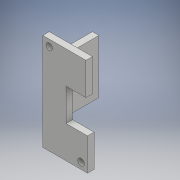
# Autodesk Inventor part: support-srf04
Saved by Autodesk Inventor 2017 (Build 210142000, 142)
## iProperties
Created: 2017-04-21
Part Number: support-srf04
Material: Generic
Document SubType Name: Modeling
Designer: franc
Density: 1 g/cm^3
Appearance: Default
Author: franc
Autodesk Inventor part; units mm, degrees
ref_plane "YZ Plane" through (0, 0, 0) normal (1, 0, 0) x (0, 1, 0)
ref_plane "XZ Plane" through (0, 0, 0) normal (0, 1, 0) x (-1, 0, 0)
ref_plane "XY Plane" through (0, 0, 0) normal (0, 0, 1) x (1, 0, 0)
sketch "Sketch1" plane through (0, 0, 0) normal (0, 1, 0) x (-1, 0, 0)
  line L0 (-9.1925, 10.3416) -> (10.8075, 10.3416)
  line L1 (10.8075, 10.3416) -> (10.8075, -34.6584)
  line L2 (10.8075, -34.6584) -> (-9.9379, -34.6584)
  line L3 (-9.9379, -34.6584) -> (-9.9379, -19.6584)
  line L4 (-9.1925, 10.3416) -> (-9.1925, -4.6584)
  line L5 (-9.1925, -4.6584) -> (0.0621, -4.6584)
  line L6 (0.0621, -4.6584) -> (0.0621, -19.6584)
  line L7 (0.0621, -19.6584) -> (-9.9379, -19.6584)
  circle A0 centre (-6.9379, -31.6584) radius 1.5
  circle A1 centre (7.8075, 7.3416) radius 1.5
  point P0 (0, 0)
  dimension "d0" = 20
  dimension "d1" = 45
  dimension "d2" = 15
  dimension "d3" = 15
  dimension "d4" = 10
  dimension "d5" = 3
  dimension "d6" = 3
  dimension "d7" = 3
  dimension "d8" = 3
  dimension "d9" = 3
  dimension "d10" = 3
  constraints: 16 end point, 6 perpendicular, 2 centre point, 1 horizontal, 1 vertical
  measures "d0" distance of L0.start L0.end
  measures "d1" distance of L0.end L1.end
  measures "d2" distance of L0.start L4.end
  measures "d3" distance of L2.end L3.end
  measures "d4" distance of L6.end L3.end
  measures "d5" distance from line of L2 A0.centre
  measures "d6" distance from line of L3 A0.centre
  measures "d7" diameter of A0
  measures "d8" distance from line of L0 A1.centre
  measures "d9" distance from line of L1 A1.centre
  measures "d10" diameter of A1
extrude "Extrusion1" add sketch "Sketch1" along normal blind 3
sketch "Sketch2" plane through (0, 3, 0) normal (0, 1, 0) x (1, 0, 0)
  line L0 (-10.8075, 34.6584) -> (-10.8075, -10.3416) projected
  line L1 (-10.8075, -0.3416) -> (-7.8075, -0.3416)
  line L2 (-7.8075, -0.3416) -> (-7.8075, 24.6584)
  line L3 (-7.8075, 24.6584) -> (-10.8075, 24.6584)
  line L4 (-10.8075, 24.6584) -> (-10.8075, -0.3416)
  line L5 (9.9379, 34.6584) -> (-10.8075, 34.6584) projected
  line L6 (-10.8075, -10.3416) -> (9.1925, -10.3416) projected
  point P0 (0, 0)
  dimension "d13" = 10
  dimension "d14" = 10
  dimension "d15" = 3
  constraints: 8 end point, 2 parallel, 1 horizontal, 1 perpendicular, 1 point on line
  measures "d13" distance between parallel lines of L5 L3
  measures "d14" distance between parallel lines of L6 L1
  measures "d15" distance of L1.start L1.end
extrude "Extrusion2" add sketch "Sketch2" along normal blind 20
sketch "Sketch3" plane through (-10.8075, 0, -34.6584) normal (-1, 0, 0) x (0, 0, 1)
  circle A0 centre (22.5, 13) radius 1.5
  line L0 (10, 23) -> (35, 23) projected
  line L1 (10, 3) -> (10, 23) projected
  point P0 (34.6584, 0)
  dimension "d18" = 10
  dimension "d19" = 12.5
  dimension "d20" = 3
  constraints: 1 centre point
  measures "d18" distance from line of L0 A0.centre
  measures "d19" distance from line of L1 A0.centre
  measures "d20" diameter of A0
extrude "Extrusion3" cut sketch "Sketch3" against normal up to surface (3 mm away)
body "Solid1"
